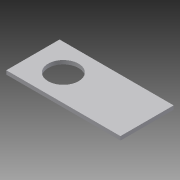
# Autodesk Inventor part: UNLHEP-14-01-P-015_PickerStrip
Saved by Autodesk Inventor 2013 (Build 170138000, 138)
## iProperties
Created: 2014-01-23
Part Number: UNLHEP-14-01-P-015_PickerStrip
Material: Allgemein
Document SubType Name: Modeling
Designer: Frank Meier
Density: 1 g/cm^3
Project: UNL Pixel Phase I
Author: Frank Meier
Autodesk Inventor part; units mm, degrees
ref_plane "YZ Plane" through (0, 0, 0) normal (1, 0, 0) x (0, 1, 0)
ref_plane "XZ Plane" through (0, 0, 0) normal (0, 1, 0) x (-1, 0, 0)
ref_plane "XY Plane" through (0, 0, 0) normal (0, 0, 1) x (1, 0, 0)
sketch "Skizze1" plane through (0, 0, 0) normal (0, 0, 1) x (1, 0, 0)
  line L0 (-7.5, -3.5) -> (7.5, -3.5)
  line L1 (7.5, -3.5) -> (7.5, 3.5)
  line L2 (7.5, 3.5) -> (-7.5, 3.5)
  line L3 (-7.5, 3.5) -> (-7.5, -3.5)
  line L4 (-7.5, -3.5) -> (7.5, 3.5) construction
  line L5 (7.5, -3.5) -> (-7.5, 3.5) construction
  point P0 (0, 0)
  dimension "d0" = 15
  dimension "d1" = 7
  constraints: 12 end point, 2 midpoint, 2 parallel, 1 horizontal, 1 perpendicular
  measures "d0" distance of L1.end L2.end
  measures "d1" distance of L0.end L1.end
extrude "Extrusion1" add sketch "Skizze1" along normal blind 0.5
hole "Bohrung1" at (-3.5, 0, 0.5) direction (0, 0, -1) diameter 4 depth 8 tip angle 118
